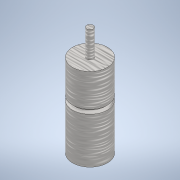
# Autodesk Inventor part: Motor
Saved by Autodesk Inventor 2022 (Build 260153000, 153)
## iProperties
Created: 2022-08-09
Part Number: Motor
Material: Generic
Document SubType Name: Modeling
Designer: Nick
Density: 3.51664 g/cm^3
Appearance: Satin Brushed
Mass: 53 g
Surface Area: 38.7247 cm^2
Volume: 15.0712 cm^3
Author: Nick
Autodesk Inventor part; units mm, degrees
ref_plane "YZ Plane" through (0, 0, 0) normal (1, 0, 0) x (0, 1, 0)
ref_plane "XZ Plane" through (0, 0, 0) normal (0, 1, 0) x (-1, 0, 0)
ref_plane "XY Plane" through (0, 0, 0) normal (0, 0, 1) x (1, 0, 0)
sketch "Sketch6" plane through (0, 0, 0) normal (0, 0, 1) x (1, 0, 0)
  line L0 (0, 0) -> (8, 0)
  line L1 (8, 0) -> (8, 38)
  line L2 (8, 38) -> (0, 38)
  line L3 (0, 38) -> (0, 0)
  line L4 (0, 38) -> (1.5, 38)
  line L5 (1.5, 38) -> (1.5, 50)
  line L6 (1.5, 50) -> (0, 50)
  line L7 (0, 50) -> (0, 38)
  line L8 (8, 23) -> (7, 22)
  line L9 (7, 22) -> (8, 21)
  dimension "d31" = 16
  dimension "d32" = 3
  dimension "d33" = 12
  dimension "d35" = 1
  dimension "d36" = 16
  dimension "d37" = 50
  constraints: 20 end point, 4 parallel, 4 perpendicular, 2 horizontal, 2 point on line
  measures "d31" diameter of L1 L3
  measures "d32" diameter of L5 L7
  measures "d33" distance of L4.end L5.end
  measures "d35" distance from line of L1 L8.end
  measures "d36" distance from line of L2 L8.end
  measures "d37" distance between parallel lines of L6 L0
revolve "Revolution2" add sketch "Sketch6" angle 360 about axis through (0, 38, 0) along (0, -1, 0) contours L3 L2 L1 L8 L9 L0 | L7 L6 L5 L2
body "Solid2"
